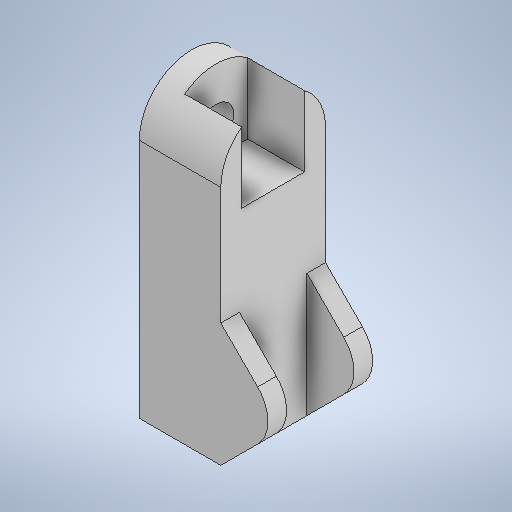
# Autodesk Inventor part: SideCameraSlider
Saved by Autodesk Inventor 2025.1 (Build 291241000, 241)
## iProperties
Created: 2026-04-27
Part Number: SideCameraSlider
Material: Generic
Document SubType Name: Modeling
Designer: User
Density: 1 g/cm^3
Appearance: Default
Author: User
## iProperties of the stored document SideCameraSlider_3DPrint.ipt
Created: 2026-04-30
Part Number: SideCameraSlider_3DPrint
Material: Generic
Document SubType Name: Modeling
Designer: User
Density: 1 g/cm^3
Appearance: Default
Author: User
Autodesk Inventor part; units mm, degrees
ref_plane "YZ Plane" through (0, 0, 0) normal (1, 0, 0) x (0, 1, 0)
ref_plane "Work Plane1" through (0, 0, 0) normal (0, 0, 1) x (1, 0, 0)
sketch "Sketch1" plane through (0, 0, 0) normal (0, 0, 1) x (1, 0, 0)
  line L0 (-12.5, 1) -> (-12.5, -7.7) projected
  line L1 (-12.5, 12) -> (-12.5, 6.5) projected
  line L2 (-12.6, 1) -> (-12.6, -7.7)
  line L3 (-12.6, 12) -> (-12.6, 9.0456)
  arc A0 (-12.5, 1) -> (-12.5, 6.5) centre (-11.5571, 3.75) ccw projected
  line L4 (-12.4, 12) -> (-12.4, 6.6366)
  arc A1 (-9.4308, 1.6236) -> (-9.4308, 5.8764) centre (-11.5571, 3.75) ccw
  line L5 (-12.4, 0.8634) -> (-12.4, -7.7)
  line L6 (-9.4308, 5.8764) -> (-12.6, 9.0456)
  line L7 (-8.6562, 5.1018) -> (-1.312, 5.1018) construction
  line L8 (-9.4308, 1.6236) -> (-12.6, -1.5456)
  line L9 (-8.3764, 2.678) -> (0.7652, 2.678) construction
  line L10 (-19.6, -14) -> (-19.6, -6.5) projected
  line L11 (-12.6, -1.5456) -> (-19.6, -1.5456)
  line L12 (-17.5, 16.8) -> (-17.5, 21.5) projected
  line L13 (-12.5, 16.8) -> (-17.5, 16.8) projected
  line L14 (-12.6, 16.7) -> (-17.5, 16.7)
  line L15 (-12.6, 12) -> (-12.6, 16.7)
  line L16 (-17.5, 16.8) -> (-17.5, 16.7)
  line L17 (-19.6, -1.5456) -> (-19.6, 21.5)
  line L18 (-19.6, -1.5456) -> (3.4456, -1.5456) construction
  line L19 (-19.6, 21.5) -> (-17.5, 21.5)
  point P0 (0, 0)
  dimension "d0" = 0.1
  dimension "d1" = 0.1
  dimension "d2" = 0.1
  dimension "d3" = 135
  dimension "d4" = 135
  dimension "d5" = 0.1
  dimension "d6" = 90
  constraints: 30 end point, 4 horizontal, 4 perpendicular, 2 parallel, 2 point on circle, 2 tangent, 1 centre point, 1 point on line
  measures "d0" distance between parallel lines of L0 L2
  measures "d1" distance between parallel lines of L1 L3
  measures "d2" radial gap between concentric circles of A0 A1
  measures "d3" angle of L7 L6
  measures "d4" angle of L8 L9
  measures "d5" distance between parallel lines of L13 L14
  measures "d6" angle of L18 L17
extrude "Extrusion1" add sketch "Sketch1" along normal blind 2
sketch "Sketch2" plane through (0, 0, 0) normal (0, 0, -1) x (-1, 0, 0)
  line L0 (19.6, -1.5456) -> (12.6, -1.5456) projected
  line L1 (12.6, 9.0456) -> (12.6, 16.7) projected
  line L2 (12.6, 16.7) -> (17.5, 16.7) projected
  line L3 (17.5, 16.7) -> (17.5, 21.5) projected
  line L4 (17.5, 21.5) -> (19.6, 21.5) projected
  line L5 (19.6, 21.5) -> (19.6, -1.5456) projected
  line L6 (12.6, -1.5456) -> (12.6, 9.0456)
  point P0 (0, 0)
  constraints: 2 end point, 1 collinear
ref_plane "Work Plane2" through (-17.5, 12.1, -5) normal (0, 0, -1) x (0, 1, 0)
extrude "Extrusion2" add sketch "Sketch2" along normal up to surface (5 mm away)
sketch "Sketch3" plane through (-12.6, -1.5456, -5) normal (0, 0, -1) x (-1, 0, 0)
  line L0 (0, 10.5912) -> (0, 18.2456) projected
  line L1 (0, 18.2456) -> (4.9, 18.2456) projected
  line L2 (4.9, 18.2456) -> (4.9, 23.0456) projected
  line L3 (4.9, 23.0456) -> (7, 23.0456) projected
  line L4 (7, 23.0456) -> (7, 0) projected
  line L5 (7, 0) -> (0, 0) projected
  line L6 (0, 0) -> (-3.1692, 3.1692) projected
  arc A0 (-3.1692, 7.422) -> (-3.1692, 3.1692) centre (-1.0429, 5.2956) ccw projected
  line L7 (-3.1692, 7.422) -> (0, 10.5912) projected
  point P0 (-12.6, 1.5456)
extrude "Extrusion3" add sketch "Sketch3" along normal blind 2
sketch "Sketch4" plane through (-19.6, -1.5456, 2) normal (-1, 0, 0) x (0, 0, 1)
  line L0 (-2, 23.0456) -> (-2, 18.3456) projected
  line L1 (-7, 18.3456) -> (-2, 18.3456) projected
  line L2 (-7, 23.0456) -> (-7, 18.3456) projected
  line L3 (-7, 23.0456) -> (-2, 23.0456) projected
  line L4 (-2, 18.3456) -> (-7, 23.0456)
  circle A0 centre (-4.5, 20.6956) radius 1.5
  circle A1 centre (-4.5, 20.6956) radius 1.4 projected
  point P0 (-2, 1.5456)
  dimension "d13" = 3
  constraints: 2 end point, 1 centre point, 1 midpoint
  measures "d13" diameter of A0
extrude "Extrusion4" cut sketch "Sketch4" against normal blind 2.75 contours A0 L4 A1 | L4 A1 A0 | A1 L4 | L4 A1
sketch "Sketch5" plane through (-19.6, -1.5456, 2) normal (-1, 0, 0) x (0, 0, 1)
  circle A0 centre (-4.5, 20.6956) radius 1.5 projected
  line L0 (0, 23.0456) -> (0, 0) projected
  circle A1 centre (-4.5, 20.6956) radius 4.5
  line L1 (0, 23.0456) -> (-9, 23.0456) projected
  point P0 (-2, 1.5456)
  point P1 (-8.3376, 23.0456)
  point P2 (-0.6624, 23.0456)
  constraints: 1 centre point, 1 coincident, 1 tangent
extrude "Extrusion5" add sketch "Sketch5" against normal up to surface (2.1 mm away) contours L1 A1 picked at (-4.7918, 23.9439)
sketch "Sketch6" plane through (-19.6, -1.5456, 2) normal (-1, 0, 0) x (0, 0, 1)
  arc A0 (-0.6624, 23.0456) -> (-8.3376, 23.0456) centre (-4.5, 20.6956) ccw projected
  line L0 (0, 23.0456) -> (0, 0) projected
  line L1 (0, 23.0456) -> (-0.6624, 23.0456) projected
  circle A1 centre (-4.5, 20.6956) radius 4.5
  line L2 (-8.3376, 23.0456) -> (-9, 23.0456) projected
  line L3 (-9, 0) -> (-9, 23.0456) projected
  point P0 (-2, 1.5456)
  point P1 (-9, 20.6956)
  point P2 (-8.3376, 23.0456)
  point P3 (0, 20.6956)
  constraints: 1 coincident, 3 other
extrude "Extrusion6" cut sketch "Sketch6" against normal blind 10 contours L1 L0 A1 | A1 L3 L2
sketch "Sketch7" plane through (-17.5, 16.7, 2) normal (1, 0, 0) x (0, 0, -1)
  line L0 (7, 4.8) -> (7, 0.1) projected
  line L1 (2, 4.8) -> (2, 0.1) projected
  line L2 (7.2, 4.8) -> (7.2, 0.1)
  line L3 (1.8, 4.8) -> (1.8, 0.1)
  arc A0 (9, 2.45) -> (0, 2.45) centre (4.5, 2.45) ccw projected
  line L4 (9, 2.45) -> (9, 0) projected
  line L5 (0, 0) -> (0, 2.45) projected
  line L6 (9, 0) -> (0, 0) projected
  line L7 (1.8, 0.1) -> (1.8, 0)
  line L8 (9, 0) -> (0, 0) projected
  line L9 (7.2, 0.1) -> (7.2, 0)
  line L10 (7.2, 4.8) -> (7.2, 6.05)
  line L11 (1.8, 4.8) -> (1.8, 6.05)
  point P0 (2, -16.7)
  point P1 (1.8, 0)
  dimension "d20" = 0.2
  dimension "d21" = 0.2
  constraints: 12 end point, 3 parallel, 2 perpendicular, 2 point on circle, 2 point on line, 1 vertical
  measures "d20" distance between parallel lines of L0 L2
  measures "d21" distance between parallel lines of L1 L3
extrude "Extrusion7" add sketch "Sketch7" along normal up to surface (4.9 mm away) contours L10 A0 L4 L6 L9 L2 | L11 L3 L7 L6 L5 A0
sketch "Sketch8" plane through (0, 0, 0) normal (0, 0, -1) x (-1, 0, 0)
  line L0 (12.6, -1.5456) -> (12.6, 9.0456) projected
  line L1 (9.4308, 5.8764) -> (12.6, 9.0456) projected
  arc A0 (9.4308, 5.8764) -> (9.4308, 1.6236) centre (11.5571, 3.75) ccw projected
  line L2 (12.6, -1.5456) -> (9.4308, 1.6236) projected
  point P0 (0, 0)
extrude "Extrusion8" cut sketch "Sketch8" against normal blind 0.4
sketch "Sketch9" plane through (-12.6, -1.5456, -5) normal (0, 0, 1) x (1, 0, 0)
  line L0 (0, 0) -> (0, 10.5912) projected
  line L1 (3.1692, 3.1692) -> (0, 0) projected
  arc A0 (3.1692, 3.1692) -> (3.1692, 7.422) centre (1.0429, 5.2956) ccw projected
  line L2 (0, 10.5912) -> (3.1692, 7.422) projected
  point P0 (12.6, 1.5456)
extrude "Extrusion9" cut sketch "Sketch9" against normal blind 0.4
body "Solid1"
